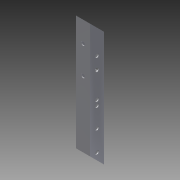
# Autodesk Inventor part: Square Tube 3
Saved by Autodesk Inventor 2013 (Build 170138000, 138)
## iProperties
Created: 2013-01-24
Part Number: Square Tube 3
Material: Aluminum 6061
Document SubType Name: Modeling
Designer: actoennies
Mass: 84.0179 g
Surface Area: 398.909 cm^2
Volume: 31.0029 cm^3
Density: 2.71 g/cm^3
Author: actoennies
Autodesk Inventor part; units mm, degrees
ref_plane "YZ Plane" through (0, 0, 0) normal (1, 0, 0) x (0, 1, 0)
ref_plane "XZ Plane" through (0, 0, 0) normal (0, 1, 0) x (-1, 0, 0)
ref_plane "XY Plane" through (0, 0, 0) normal (0, 0, 1) x (1, 0, 0)
sketch "Sketch1" plane through (0, 0, 0) normal (0, 1, 0) x (-1, 0, 0)
  line L0 (0, 0) -> (25.4, 0)
  line L1 (25.4, 0) -> (25.4, 25.4)
  line L2 (25.4, 25.4) -> (0, 25.4)
  line L3 (0, 25.4) -> (0, 0)
  line L4 (1.5875, 23.8125) -> (23.8125, 23.8125)
  line L5 (23.8125, 23.8125) -> (23.8125, 1.5875)
  line L6 (23.8125, 1.5875) -> (1.5875, 1.5875)
  line L7 (1.5875, 1.5875) -> (1.5875, 23.8125)
  dimension "d0" = 25.4
  dimension "d2" = 25.4
  dimension "d3" = 1.5875
  constraints: 16 end point, 4 parallel, 2 perpendicular, 1 horizontal, 3 other
  measures "d0" distance of L1.end L2.end
  measures "d2" distance of L0.end L1.end
  measures "d3" distance between parallel lines of L2 L4
extrude "Extrusion1" add sketch "Sketch1" along normal blind 254
sketch "Sketch2" plane through (-25.4, 0, 0) normal (-1, 0, 0) x (0, 0, 1)
  line L0 (0, 254) -> (25.4, 254) projected
  line L1 (0, 0) -> (0, 254) projected
  line L2 (25.4, 0) -> (25.4, 254) projected
  line L3 (25.4, 234.95) -> (0, 209.55)
  point P0 (0, 228.6)
  dimension "d6" = 25.4
  dimension "d13" = 25.4
  dimension "d14" = 19.05
  constraints: 3 point on line, 2 end point
  measures "d6" distance of point (0, 228.6) L0.start
  measures "d13" horizontal distance of L3.end L3.start
  measures "d14" distance from line of L0 L3.start
extrude "Extrusion2" cut sketch "Sketch2" against normal blind 25.4
sketch "Sketch3" plane through (-25.4, 0, 0) normal (-1, 0, 0) x (0, 0, 1)
  line L0 (25.4, 254) -> (0, 228.6) projected
  line L1 (0, 0) -> (25.4, 0) projected
  line L2 (25.4, 0) -> (25.4, 234.95) projected
  line L3 (0, 0) -> (25.4, 25.4)
  constraints: 2 end point, 1 parallel, 1 point on line
extrude "Extrusion3" cut sketch "Sketch3" against normal blind 25.4
sketch "Sketch4" plane through (-25.4, 25.4, 25.4) normal (-1, 0, 0) x (0, 0, 1)
  circle A0 centre (-12.7, 38.1) radius 3.3782 projected
  circle A1 centre (-12.7, 0) radius 3.3782 projected
extrude "Extrusion4" cut sketch "Sketch4" against normal blind 25.4
sketch "Sketch5" plane through (0, 209.55, 0) normal (0, 0, -1) x (-1, 0, 0)
  circle A0 centre (12.7, -12.7) radius 3.3782 projected
  circle A1 centre (12.7, -63.5) radius 3.3782 projected
extrude "Extrusion5" cut sketch "Sketch5" against normal blind 25.4
sketch "Sketch6" plane through (0, 0, 0) normal (1, 0, 0) x (0, 0, -1)
  circle A0 centre (-12.7, 177.8) radius 3.3782 projected
  circle A1 centre (-12.7, 155.575) radius 3.3782 projected
extrude "Extrusion6" cut sketch "Sketch6" against normal blind 25.4
sketch "Sketch7" plane through (-25.4, 25.4, 25.4) normal (-1, 0, 0) x (0, 0, 1)
  circle A0 centre (-12.7, 83.1396) radius 3.3782 projected
  circle A1 centre (-12.7, 73.6146) radius 3.3782 projected
extrude "Extrusion7" cut sketch "Sketch7" against normal blind 25.4
body "Solid1"
